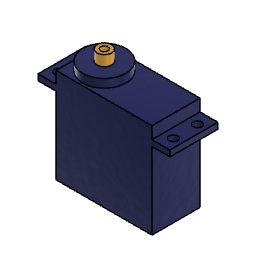
SCS125舵机 v2 (Autodesk Fusion 360 design; units mm, degrees)
Autodesk Fusion 360 part; units mm, degrees
sketch "草图1" plane through (0, 0, 0) normal (0, 0, 1) x (1, 0, 0)
  line L0 (20, -10) -> (-20, -10)
  line L1 (-20, -10) -> (-20, 10)
  line L2 (-20, 10) -> (20, 10)
  line L3 (20, 10) -> (20, -10)
  line L4 (20, -10) -> (-20, 10) construction
  line L5 (-20, -10) -> (20, 10) construction
  dimension "d1" = 20
  dimension "d2" = 40
  constraint horizontal L0
  constraint perpendicular L0 L1
  constraint parallel L0 L2
  constraint parallel L1 L3
  constraint coincident L4 origin
  constraint coincident L5 origin
  measures "d1" distance of L0.end L1.end
  measures "d2" distance of L1.end L2.end
extrude "拉伸1" add sketch "草图1" along normal blind 32 makes body 1
sketch "草图2" plane through (0, 0, 32) normal (0, 0, 1) x (-1, 0, 0)
  line L0 (-20, -10) -> (20, -10)
  line L1 (20, -10) -> (20, 10)
  line L2 (20, 10) -> (-20, 10)
  line L3 (-20, 10) -> (-20, -10)
  line L4 (-27.5, 10) -> (27.5, 10)
  line L5 (27.5, 10) -> (27.5, -10)
  line L6 (27.5, -10) -> (-27.5, -10)
  line L7 (-27.5, -10) -> (-27.5, 10)
  line L8 (-27.5, 10) -> (27.5, -10) construction
  line L9 (27.5, 10) -> (-27.5, -10) construction
  line L10 (34, 0) -> (-45, 0)
  line L11 (0, -20) -> (0, 28)
  circle A0 centre (24, -5) radius 1.75
  circle A1 centre (-24, -5) radius 1.75
  circle A2 centre (24, 5) radius 1.75
  circle A3 centre (-24, 5) radius 1.75
  dimension "d5" = 20
  dimension "d6" = 55
  dimension "d7" = 3.5
  dimension "d8" = 48
  dimension "d9" = 10
  constraint horizontal L4
  constraint perpendicular L4 L5
  constraint parallel L4 L6
  constraint parallel L5 L7
  constraint coincident L8 origin
  constraint coincident L9 origin
  constraint perpendicular L5 L10
  constraint perpendicular L6 L11
  constraint symmetric L4 L6 L10
  constraint symmetric L11 A0 A1
  constraint symmetric L10 A0 A2
  constraint symmetric L10 A1 A3
  measures "d5" distance of L4.end L5.end
  measures "d6" distance of L5.end L6.end
  measures "d7" diameter of A0
  measures "d8" distance of A0.centre A1.centre
  measures "d9" distance of A0.centre A2.centre
extrude "拉伸2" add sketch "草图2" along normal blind 2.5 bodies 1
sketch "草图4" plane through (0, 0, 34.5) normal (0, 0, 1) x (-1, 0, 0)
  circle A0 centre (24, 5) radius 1.75
  circle A1 centre (24, -5) radius 1.75
  circle A2 centre (-24, 5) radius 1.75
  circle A3 centre (-24, -5) radius 1.75
  line L0 (-27.5, -10) -> (27.5, -10)
  line L1 (27.5, -10) -> (27.5, 10)
  line L2 (27.5, 10) -> (-27.5, 10)
  line L3 (-27.5, 10) -> (-27.5, -10)
  line L4 (-20, 10) -> (20, 10)
  line L5 (20, 10) -> (20, -10)
  line L6 (20, -10) -> (-20, -10)
  line L7 (-20, -10) -> (-20, 10)
  line L8 (-20, 10) -> (20, -10) construction
  line L9 (20, 10) -> (-20, -10) construction
  dimension "d12" = 20
  dimension "d13" = 40
  constraint horizontal L4
  constraint perpendicular L4 L5
  constraint parallel L4 L6
  constraint parallel L5 L7
  constraint coincident L8 origin
  constraint coincident L9 origin
  measures "d12" distance of L4.end L5.end
  measures "d13" distance of L5.end L6.end
extrude "拉伸3" add sketch "草图4" along normal blind 5 contours L0 L2 L4 L5 L6 L7 bodies 1
sketch "草图5" plane through (0, 0, 39.5) normal (0, 0, 1) x (-1, 0, 0)
  line L0 (-20, -10) -> (20, -10)
  line L1 (20, -10) -> (20, 10)
  line L2 (20, 10) -> (-20, 10)
  line L3 (-20, 10) -> (-20, -10)
  line L4 (-20, -10) -> (-20, 10)
  line L5 (-20, 10) -> (-27.5, 10)
  line L6 (-27.5, 10) -> (-27.5, -10)
  line L7 (-27.5, -10) -> (-20, -10)
  circle A0 centre (-24, 5) radius 1.75
  circle A1 centre (-24, -5) radius 1.75
  line L8 (20, 10) -> (20, -10)
  line L9 (20, -10) -> (27.5, -10)
  line L10 (27.5, -10) -> (27.5, 10)
  line L11 (27.5, 10) -> (20, 10)
  circle A2 centre (24, -5) radius 1.75
  circle A3 centre (24, 5) radius 1.75
  circle A4 centre (9.86, 0) radius 9
  dimension "d16" = 33.86
  dimension "d17" = 18
  measures "d16" horizontal distance of A1.centre A4.centre
  measures "d17" diameter of A4
extrude "拉伸4" add sketch "草图5" along normal blind 3.5 contours A4 bodies 1
sketch "草图6" plane through (0, 0, 43) normal (0, 0, 1) x (-1, 0, 0)
  circle A0 centre (9.86, 0) radius 9
  circle A1 centre (9.86, 0) radius 3
  circle A2 centre (9.86, 0) radius 1.5
  dimension "d20" = 6
  dimension "d21" = 3
  constraint concentric A0 A1
  constraint concentric A1 A2
  measures "d20" diameter of A1
  measures "d21" diameter of A2
extrude "拉伸5" add sketch "草图6" along normal blind 4.38 separate body contours A1 makes body 2
copy_body "实体->零部件1" bodies 1 removing the originals makes body 3 in component "Component'"
copy_body "实体->零部件2" bodies 2 removing the originals makes body 4 in component "Component''"
component "Component'" placed x (1, 0, 0) y (0, 1, 0) z (0, 0, 1) at (0, 0, 0)
component "Component''" placed x (1, 0, 0) y (0, 1, 0) z (0, 0, 1) at (0, 0, 0)
